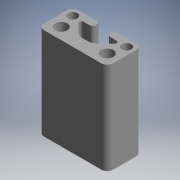
# Autodesk Inventor part: 1575-2-CL
Saved by Autodesk Inventor 2017.3 (Build 213256000, 256)
## iProperties
Part Number: 1575-2-CL
Material: Generic
Catalog Web Link: www.cadenas.de
Description: 1575, 1575-Black-FB-T-Slotted Profile - 15 Series
Vendor: 8020
Document SubType Name: Modeling
Designer: partserver
Manufacturer: 8020
Mass: 22.7861 g
Surface Area: 120.928 cm^2
Volume: 22.7861 cm^3
Density: 1 g/cm^3
Appearance: PSOLRGB-191-191-191
Category: PARTsolutions
Company: 8020
Title: 1575-2
Author: Cadenas PARTsolutions
Comments: T-Slotted Profile - 15 Series
PSOL_IDENT_0: {$CADENAS_DATA\23d-libs\8020\inch\profiles\15_series\1575.prj},180 {VTYP=3D},{NB=1575-2-CL},{LINA=15
PSOL_IDENT_1: 75-2},{NN=1575, 1575-Black-FB},{DATE=31.07.2020 09:21:23},{GEOMDATE=09.02.2018 15:52:48},{VERSION=},
PSOL_IDENT_2: {LINEID=10},{WBVAR=FINISH,LS,L},{WBNUMERIC=L}  {NB=1575-2-CL},{LINA=1575-2},{KT=DUMMY},{PN=1575-2},{
PSOL_IDENT_3: SERIES=1575},{MAT=6105-T5 Aluminum},{FINISH=CA},{LS=-CL},{L=2.000},{LALG=[1:145/0.005]},{W=.7997},{M
PSOL_IDENT_4: IX=.0380},{MIY=.1470},{EA=.6870},{CLR=.75,.75,.75}
NB: 1575-2-CL
NN: 1575, 1575-Black-FB
NT: T-Slotted Profile - 15 Series
NBSYN: $PN.$LS.
LINA: 1575-2
CATALOG: 80/20
PN: 1575-2
SERIES: 1575
MAT: 6105-T5 Aluminum
FINISH: Clear Anodize
LS: Custom Length
L: 2
W: .7997
MIX: .0380
MIY: .1470
EA: .6870
SUPPLIER: 8020
ARTICLENO: 1575-2-CL
BOMINFO: 1575-2
CREATOR: CADENAS GmbH
Autodesk Inventor part; units mm, degrees
ref_plane "YZ Plane" through (0, 0, 0) normal (1, 0, 0) x (0, 1, 0)
ref_plane "XZ Plane" through (0, 0, 0) normal (0, 1, 0) x (-1, 0, 0)
ref_plane "XY Plane" through (0, 0, 0) normal (0, 0, 1) x (1, 0, 0)
sketch "Sketch_1" plane through (0, 0, 0) normal (0, 0, 1) x (1, 0, 0)
  arc A0 (-19.05, 3.175) -> (-15.875, 0) centre (-15.875, 3.175) ccw
  line L0 (-15.875, 0) -> (15.875, 0)
  arc A1 (15.875, 0) -> (19.05, 3.175) centre (15.875, 3.175) ccw
  line L1 (19.05, 3.175) -> (19.05, 15.875)
  arc A2 (19.05, 15.875) -> (15.875, 19.05) centre (15.875, 15.875) ccw
  line L2 (15.875, 19.05) -> (5.6388, 19.05)
  arc A3 (5.6388, 19.05) -> (4.064, 17.4752) centre (5.6388, 17.4752) ccw
  line L3 (4.064, 17.4752) -> (4.064, 16.5608)
  arc A4 (4.064, 16.5608) -> (5.6388, 14.986) centre (5.6388, 16.5608) ccw
  line L4 (5.6388, 14.986) -> (9.398, 14.986)
  arc A5 (10.287, 14.097) -> (9.398, 14.986) centre (9.398, 14.097) ccw
  line L5 (10.287, 14.097) -> (10.287, 13.7794)
  arc A6 (10.0266, 13.1508) -> (10.287, 13.7794) centre (9.398, 13.7794) ccw
  line L6 (10.0266, 13.1508) -> (5.125, 8.2492)
  arc A7 (1.7664, 6.858) -> (5.125, 8.2492) centre (1.7664, 11.6078) ccw
  line L7 (1.7664, 6.858) -> (-1.7664, 6.858)
  arc A8 (-5.125, 8.2492) -> (-1.7664, 6.858) centre (-1.7664, 11.6078) ccw
  line L8 (-5.125, 8.2492) -> (-10.0266, 13.1508)
  arc A9 (-10.287, 13.7794) -> (-10.0266, 13.1508) centre (-9.398, 13.7794) ccw
  line L9 (-10.287, 13.7794) -> (-10.287, 14.097)
  arc A10 (-9.398, 14.986) -> (-10.287, 14.097) centre (-9.398, 14.097) ccw
  line L10 (-9.398, 14.986) -> (-5.6388, 14.986)
  arc A11 (-5.6388, 14.986) -> (-4.064, 16.5608) centre (-5.6388, 16.5608) ccw
  line L11 (-4.064, 16.5608) -> (-4.064, 17.4752)
  arc A12 (-4.064, 17.4752) -> (-5.6388, 19.05) centre (-5.6388, 17.4752) ccw
  line L12 (-5.6388, 19.05) -> (-15.875, 19.05)
  arc A13 (-15.875, 19.05) -> (-19.05, 15.875) centre (-15.875, 15.875) ccw
  line L13 (-19.05, 15.875) -> (-19.05, 3.175)
  circle A14 centre (14.8488, 14.8014) radius 2.5527
  circle A15 centre (12.7, 6.35) radius 3.3274
  circle A16 centre (-12.7, 6.35) radius 3.3274
  circle A17 centre (-14.8488, 14.8014) radius 2.5527
  constraints: 28 end point, 28 point on circle, 18 centre point
extrude "Extrusion1" add sketch "Sketch_1" against normal blind 50.8
body "Solid1"
